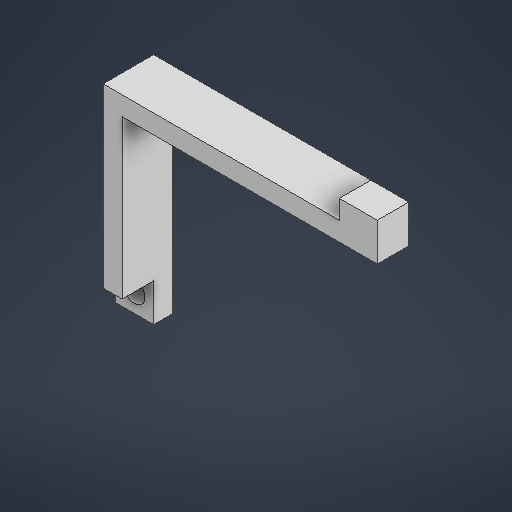
# Autodesk Inventor part: leftbmw2
Saved by Autodesk Inventor 2026.2 (Build 302298010, 298A)
## iProperties
Created: 2026-09-07
Part Number: leftbmw2
Material: Generic
Document SubType Name: Modeling
Designer: karol
Density: 1 g/cm^3
Appearance: Default
Author: karol
Autodesk Inventor part; units mm, degrees
ref_plane "YZ Plane" through (0, 0, 0) normal (1, 0, 0) x (0, 1, 0)
ref_plane "XZ Plane" through (0, 0, 0) normal (0, 1, 0) x (-1, 0, 0)
ref_plane "XY Plane" through (0, 0, 0) normal (0, 0, 1) x (1, 0, 0)
sketch "Sketch1" plane through (0, 0, 0) normal (0, 0, 1) x (1, 0, 0)
  line L0 (-58, -60) -> (-60, -60) projected
  line L1 (-60, -60) -> (-60, -39.5) projected
  line L2 (-60, -39.5) -> (-58, -39.5) projected
  line L3 (-58, -39.5) -> (-58, -60) projected
  line L4 (49.6, 30) -> (51.6, 30) projected
  line L5 (51.6, 30) -> (51.6, 9.5) projected
  line L6 (51.6, 9.5) -> (49.6, 9.5) projected
  line L7 (49.6, 9.5) -> (49.6, 30) projected
  line L8 (-58, 39.5) -> (-60, 39.5) projected
  line L9 (-60, 39.5) -> (-60, 60) projected
  line L10 (-60, 60) -> (-58, 60) projected
  line L11 (-58, 60) -> (-58, 39.5) projected
  line L12 (-21.6, -39.5) -> (-19.6, -39.5) projected
  line L13 (-19.6, -39.5) -> (-19.6, -60) projected
  line L14 (-19.6, -60) -> (-21.6, -60) projected
  line L15 (-21.6, -60) -> (-21.6, -39.5) projected
  line L16 (51.6, -30) -> (49.6, -30) projected
  line L17 (49.6, -30) -> (49.6, -9.5) projected
  line L18 (49.6, -9.5) -> (51.6, -9.5) projected
  line L19 (51.6, -9.5) -> (51.6, -30) projected
  line L20 (-21.6, 60) -> (-19.6, 60) projected
  line L21 (-19.6, 60) -> (-19.6, 39.5) projected
  line L22 (-19.6, 39.5) -> (-21.6, 39.5) projected
  line L23 (-21.6, 39.5) -> (-21.6, 60) projected
  line L24 (90, -35) -> (90, 35) projected
  line L25 (90, 35) -> (49.6, 35) projected
  line L26 (49.6, 35) -> (49.6, 60) projected
  line L27 (49.6, 60) -> (90, 60) projected
  line L28 (90, 60) -> (90, 90) projected
  line L29 (90, 90) -> (-19.6, 90) projected
  line L30 (-19.6, 90) -> (-19.6, 65) projected
  line L31 (-19.6, 65) -> (-60, 65) projected
  line L32 (-60, 65) -> (-60, 90) projected
  line L33 (-60, 90) -> (-90, 90) projected
  line L34 (-90, 90) -> (-90, -90) projected
  line L35 (-90, -90) -> (-60, -90) projected
  line L36 (-60, -90) -> (-60, -65) projected
  line L37 (-60, -65) -> (-19.6, -65) projected
  line L38 (-19.6, -65) -> (-19.6, -90) projected
  line L39 (-19.6, -90) -> (90, -90) projected
  line L40 (90, -90) -> (90, -60) projected
  line L41 (90, -60) -> (49.6, -60) projected
  line L42 (49.6, -60) -> (49.6, -35) projected
  line L43 (49.6, -35) -> (90, -35) projected
  line L44 (86, -32) -> (73.8, -32) projected
  line L45 (73.8, -32) -> (73.8, -7.5) projected
  line L46 (73.8, -7.5) -> (86, -7.5) projected
  line L47 (86, -7.5) -> (86, -32) projected
  line L48 (65.8, -32) -> (53.6, -32) projected
  line L49 (53.6, -32) -> (53.6, -7.5) projected
  line L50 (53.6, -7.5) -> (65.8, -7.5) projected
  line L51 (65.8, -7.5) -> (65.8, -32) projected
  line L52 (86, -86) -> (70.6, -86) projected
  line L53 (70.6, -86) -> (70.6, -69.8) projected
  line L54 (70.6, -69.8) -> (86, -69.8) projected
  line L55 (86, -69.8) -> (86, -86) projected
  line L56 (86, 86) -> (86, 69.8) projected
  line L57 (86, 69.8) -> (70.6, 69.8) projected
  line L58 (70.6, 69.8) -> (70.6, 86) projected
  line L59 (70.6, 86) -> (86, 86) projected
  line L60 (73.8, 32) -> (86, 32) projected
  line L61 (86, 32) -> (86, 7.5) projected
  line L62 (86, 7.5) -> (73.8, 7.5) projected
  line L63 (73.8, 7.5) -> (73.8, 32) projected
  line L64 (65.8, 32) -> (65.8, 7.5) projected
  line L65 (65.8, 7.5) -> (53.6, 7.5) projected
  line L66 (53.6, 7.5) -> (53.6, 32) projected
  line L67 (53.6, 32) -> (65.8, 32) projected
  line L68 (-69.6, -87) -> (-85, -87) projected
  line L69 (-85, -87) -> (-85, -70.8) projected
  line L70 (-85, -70.8) -> (-69.6, -70.8) projected
  line L71 (-69.6, -70.8) -> (-69.6, -87) projected
  line L72 (-56, -62) -> (-56, -37.5) projected
  line L73 (-56, -37.5) -> (-43.8, -37.5) projected
  line L74 (-43.8, -37.5) -> (-43.8, -62) projected
  line L75 (-43.8, -62) -> (-56, -62) projected
  line L76 (-56, 62) -> (-43.8, 62) projected
  line L77 (-43.8, 62) -> (-43.8, 37.5) projected
  line L78 (-43.8, 37.5) -> (-56, 37.5) projected
  line L79 (-56, 37.5) -> (-56, 62) projected
  line L80 (-23.6, 62) -> (-23.6, 37.5) projected
  line L81 (-23.6, 37.5) -> (-35.8, 37.5) projected
  line L82 (-35.8, 37.5) -> (-35.8, 62) projected
  line L83 (-35.8, 62) -> (-23.6, 62) projected
  line L84 (-23.6, -62) -> (-35.8, -62) projected
  line L85 (-35.8, -62) -> (-35.8, -37.5) projected
  line L86 (-35.8, -37.5) -> (-23.6, -37.5) projected
  line L87 (-23.6, -37.5) -> (-23.6, -62) projected
  line L88 (-85, 87) -> (-69.6, 87) projected
  line L89 (-69.6, 87) -> (-69.6, 70.8) projected
  line L90 (-69.6, 70.8) -> (-85, 70.8) projected
  line L91 (-85, 70.8) -> (-85, 87) projected
  line L92 (90, -35) -> (43.6, -35) projected
  line L93 (90, -35) -> (90, 35) projected
  line L94 (90, 35) -> (43.6, 35) projected
  line L95 (43.6, 29) -> (43.6, 35) projected
  line L96 (49.6, 29) -> (43.6, 29) projected
  line L97 (49.6, 29) -> (49.6, 32) projected
  line L98 (49.6, 32) -> (87, 32) projected
  line L99 (87, 32) -> (87, -32) projected
  line L100 (87, -32) -> (49.6, -32) projected
  line L101 (49.6, -32) -> (49.6, -29) projected
  line L102 (49.6, -29) -> (43.6, -29) projected
  line L103 (43.6, -35) -> (43.6, -29) projected
  line L104 (49.6, 35) -> (46.6, 35)
  line L105 (46.6, 35) -> (46.6, 60)
  line L106 (46.6, 60) -> (49.6, 60)
  line L107 (49.6, 60) -> (49.6, 35)
  line L108 (49.6, 35) -> (43.6, 35)
  line L109 (43.6, 35) -> (43.6, 29)
  line L110 (43.6, 29) -> (49.6, 29)
  line L111 (49.6, 29) -> (49.6, 35)
  line L112 (46.6, 60) -> (90, 60)
  line L113 (90, 60) -> (90, 63)
  line L114 (90, 63) -> (46.6, 63)
  line L115 (46.6, 63) -> (46.6, 60)
  point P0 (0, 0)
  dimension "d0" = 3
  dimension "d1" = 3
  constraints: 24 end point, 6 parallel, 3 horizontal, 3 perpendicular, 2 point on line
  measures "d0" distance of L105.end L106.end
  measures "d1" distance of L113.end L112.end
extrude "Extrusion1" add sketch "Sketch1" along normal blind 8 contours L94 L105 L106 L26 | L106 L115 L114 L28 L27
ref_plane "Work Plane1" through (0, 0, 0) normal (0, 0, 1) x (1, 0, 0)
sketch "Sketch2" plane through (0, 0, 0) normal (0, 0, 1) x (1, 0, 0)
  line L0 (90, -35) -> (43.6, -35) projected
  line L1 (90, -35) -> (90, 35) projected
  line L2 (90, 35) -> (43.6, 35) projected
  line L3 (43.6, 29) -> (43.6, 35) projected
  line L4 (49.6, 29) -> (43.6, 29) projected
  line L5 (49.6, 29) -> (49.6, 32) projected
  line L6 (49.6, 32) -> (87, 32) projected
  line L7 (87, 32) -> (87, -32) projected
  line L8 (87, -32) -> (49.6, -32) projected
  line L9 (49.6, -32) -> (49.6, -29) projected
  line L10 (49.6, -29) -> (43.6, -29) projected
  line L11 (43.6, -35) -> (43.6, -29) projected
  line L12 (46.6, 35) -> (49.6, 35) projected
  line L13 (49.6, 35) -> (43.6, 35)
  line L14 (43.6, 35) -> (43.6, 29)
  line L15 (43.6, 29) -> (49.6, 29)
  line L16 (49.6, 29) -> (49.6, 35)
  point P0 (0, 0)
  constraints: 8 end point, 2 parallel, 1 horizontal, 1 perpendicular
extrude "Extrusion2" add sketch "Sketch2" along normal blind 3 contours L16 L5 L4 L3 L2
sketch "Sketch3" plane through (0, 0, 0) normal (0, 0, -1) x (-1, 0, 0)
  line L0 (-43.6, 29) -> (-49.6, 29) projected
  line L1 (-49.6, 29) -> (-49.6, 35) projected
  line L2 (-43.6, 29) -> (-49.6, 35)
  line L3 (-46.6, 35) -> (-43.6, 35) projected
  line L4 (-49.6, 29) -> (-43.6, 35)
  circle A0 centre (-46.6, 32) radius 1.65
  point P0 (0, 0)
  dimension "d6" = 3.3
  constraints: 4 end point, 1 centre point, 1 midpoint
  measures "d6" diameter of A0
extrude "Extrusion3" cut sketch "Sketch3" against normal blind 3 contours A0 L4 L2 | L2 L4 A0 | A0 L2 L4 | L2 A0 L4
sketch "Sketch7" plane through (46.6, 63, 0) normal (0, 1, 0) x (1, 0, 0)
  line L0 (3, -8) -> (43.4, -8) projected
  line L1 (43.4, -8) -> (37.4, -8)
  line L2 (37.4, -8) -> (37.4, -3)
  line L3 (37.4, -3) -> (43.4, -3)
  line L4 (43.4, -3) -> (43.4, -8)
  point P0 (-46.6, 0)
  dimension "d19" = 6
  dimension "d20" = 5
  constraints: 8 end point, 2 parallel, 1 horizontal, 1 perpendicular
  measures "d19" distance of L2.end L3.end
  measures "d20" distance of L1.end L2.end
extrude "Extrusion7" add sketch "Sketch7" along normal blind 3
sketch "Sketch8" plane through (46.6, 63, 0) normal (0, 1, 0) x (1, 0, 0)
  line L0 (3, 0) -> (43.4, 0) projected
  line L1 (37.4, -8) -> (37.4, -3) projected
  line L2 (43.4, 0) -> (37.4, 0)
  line L3 (37.4, 0) -> (37.4, -3)
  line L4 (37.4, -3) -> (43.4, -3)
  line L5 (43.4, -3) -> (43.4, 0)
  point P0 (-46.6, 0)
  constraints: 8 end point, 2 parallel, 1 horizontal, 1 perpendicular
extrude "Extrusion8" cut sketch "Sketch8" against normal blind 3
sketch "Sketch9" plane through (90, 66, 3) normal (0, 0, -1) x (-1, 0, 0)
  line L0 (0, -6) -> (0, 0) projected
  line L1 (6, -3) -> (6, -6) projected
  line L2 (0, 0) -> (6, -6)
  line L3 (6, -6) -> (6, 0)
  line L4 (6, 0) -> (0, -6)
  circle A0 centre (3, -3) radius 2
  point P0 (90, -66)
  dimension "d25" = 4
  constraints: 6 end point, 1 centre point, 1 collinear, 1 midpoint, 1 perpendicular
  measures "d25" diameter of A0
extrude "Extrusion9" cut sketch "Sketch9" against normal blind 4 contours A0 L2 L4 | L4 L2 A0 | A0 L4 L2 | L4 A0 L2
body "Solid1"
